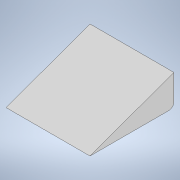
# Autodesk Inventor part: 20Grad_Winkelreduktion
Saved by Autodesk Inventor 2020 (Build 240168000, 168)
## iProperties
Created: 2020-07-10
Part Number: 20Grad_Winkelreduktion
Material: Generisch
Document SubType Name: Modeling
Designer: MartinDJay
Density: 1 g/cm^3
Appearance: Vorgabe
Author: MartinDJay
Autodesk Inventor part; units mm, degrees
ref_plane "YZ Plane" through (0, 0, 0) normal (1, 0, 0) x (0, 1, 0)
ref_plane "XZ Plane" through (0, 0, 0) normal (0, 1, 0) x (-1, 0, 0)
ref_plane "XY Plane" through (0, 0, 0) normal (0, 0, 1) x (1, 0, 0)
sketch "Skizze1" plane through (0, 0, 0) normal (1, 0, 0) x (0, 1, 0)
  line L0 (0, 17) -> (0, -17)
  line L1 (0, -17) -> (12.375, -17)
  line L2 (12.375, -17) -> (0, 17)
  point P0 (0, 0)
  point P1 (0, 0)
  dimension "d0" = 34
  dimension "d1" = 20
  constraints: 6 end point, 1 coincident, 1 midpoint, 1 perpendicular, 1 vertical
  measures "d0" distance of L0.start L0.end
  measures "d1" angle of L2 L0
extrude "Extrusion1" add sketch "Skizze1" along normal mid plane 34
fillet "Rundung1" radius 2 1 edges at (0, 0, -17)
